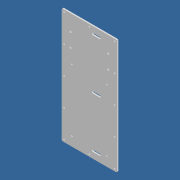
# Autodesk Inventor part: Contorller_Mount
Saved by Autodesk Inventor 2020 (Build 240168000, 168)
## iProperties
Created: 2021-07-15
Part Number: Contorller_Mount
Material: 一般
Document SubType Name: Modeling
Designer: ken113
Density: 1 g/cm^3
Appearance: 既定
Author: ken113
Autodesk Inventor part; units mm, degrees
ref_plane "YZ Plane" through (0, 0, 0) normal (1, 0, 0) x (0, 1, 0)
ref_plane "XZ Plane" through (0, 0, 0) normal (0, 1, 0) x (-1, 0, 0)
ref_plane "XY Plane" through (0, 0, 0) normal (0, 0, 1) x (1, 0, 0)
sketch "スケッチ1" plane through (0, 0, 0) normal (0, 0, 1) x (1, 0, 0)
  line L0 (50, -115) -> (-50, -115)
  line L1 (-50, -115) -> (-50, 115)
  line L2 (-50, 115) -> (50, 115)
  line L3 (50, 115) -> (50, -115)
  line L4 (50, -115) -> (-50, 115) construction
  line L5 (-50, -115) -> (50, 115) construction
  point P0 (0, 0)
  dimension "d0" = 230
  dimension "d1" = 100
  constraints: 12 end point, 2 midpoint, 2 parallel, 1 horizontal, 1 perpendicular
  measures "d0" distance of L0.end L1.end
  measures "d1" distance of L1.end L2.end
extrude "押し出し1" add sketch "スケッチ1" along normal blind 3
sketch "スケッチ2" plane through (0, 0, 3) normal (0, 0, 1) x (1, 0, 0)
  line L0 (38, -105) -> (-38, -105)
  line L1 (-38, -105) -> (-38, 30)
  line L2 (-38, 30) -> (38, 30)
  line L3 (38, 30) -> (38, -105)
  line L4 (38, -105) -> (-38, 30) construction
  line L5 (-38, -105) -> (38, 30) construction
  line L6 (-50, -115) -> (50, -115) projected
  point P0 (0, 0)
  point P1 (0, -37.5)
  point P2 (0, -37.5)
  dimension "d4" = 76
  dimension "d5" = 135
  dimension "d6" = 10
  constraints: 12 end point, 3 midpoint, 2 parallel, 1 horizontal, 1 perpendicular, 1 vertical alignment
  measures "d4" distance of L1.end L2.end
  measures "d5" distance of L2.end L0.start
  measures "d6" distance between parallel lines of L0 L6
hole "穴1" at (-38, -105, 3) at (38, -105, 3) at (38, 30, 3) at (-38, 30, 3) direction (0, 0, -1) diameter 3.2 end through all
sketch "スケッチ3" plane through (0, 0, 3) normal (0, 0, 1) x (1, 0, 0)
  line L0 (41, 60) -> (-41, 60)
  line L1 (-41, 60) -> (-41, 90)
  line L2 (-41, 90) -> (41, 90)
  line L3 (41, 90) -> (41, 60)
  line L4 (41, 60) -> (-41, 90) construction
  line L5 (-41, 60) -> (41, 90) construction
  circle A0 centre (-38, 30) radius 1.6 projected
  point P0 (0, 0)
  point P1 (0, 75)
  dimension "d14" = 82
  dimension "d15" = 30
  dimension "d16" = 30
  constraints: 12 end point, 2 midpoint, 2 parallel, 1 horizontal, 1 perpendicular
  measures "d14" distance of L1.end L2.end
  measures "d15" distance of L2.end L0.start
  measures "d16" distance from line of L0 A0.centre
hole "穴2" at (-41, 60, 3) at (41, 60, 3) at (41, 90, 3) at (-41, 90, 3) direction (0, 0, -1) diameter 4.2 end through all
sketch "スケッチ4" plane through (0, 0, 3) normal (0, 0, 1) x (1, 0, 0)
  circle A0 centre (41, 90) radius 2.1 projected
  circle A1 centre (-41, 60) radius 2.1 projected
  circle A2 centre (41, 60) radius 2.1 projected
  circle A3 centre (-41, 90) radius 2.1 projected
  circle A4 centre (38, 30) radius 1.6 projected
  circle A5 centre (-38, -105) radius 1.6 projected
  circle A6 centre (38, -105) radius 1.6 projected
  circle A7 centre (-38, 30) radius 1.6 projected
  line L0 (50, 115) -> (-50, 115) projected
  line L1 (-50, 115) -> (-50, -115) projected
  line L2 (-50, -115) -> (50, -115) projected
  line L3 (50, -115) -> (50, 115) projected
  line L4 (-60, -125) -> (-60, 125)
  line L5 (-60, 125) -> (60, 125)
  line L6 (60, 125) -> (60, -125)
  line L7 (60, -125) -> (-60, -125)
  point P0 (0, 0)
  dimension "d24" = 10
  constraints: 8 end point, 3 other
  measures "d24" distance between parallel lines of L1 L4
extrude "押し出し2" add sketch "スケッチ4" against normal up to surface (3 mm away) contours L4 L5 L6 L7
sketch "スケッチ5" plane through (0, 0, 3) normal (0, 0, 1) x (1, 0, 0)
  line L0 (60, 125) -> (-60, 125) projected
  line L1 (-60, 125) -> (-60, -125) projected
  line L2 (-60, -125) -> (60, -125) projected
  line L3 (60, -125) -> (60, 125) projected
  circle A0 centre (41, 90) radius 2.1 projected
  circle A1 centre (-41, 60) radius 2.1 projected
  circle A2 centre (41, 60) radius 2.1 projected
  circle A3 centre (-41, 90) radius 2.1 projected
  circle A4 centre (38, 30) radius 1.6 projected
  circle A5 centre (-38, -105) radius 1.6 projected
  circle A6 centre (38, -105) radius 1.6 projected
  circle A7 centre (-38, 30) radius 1.6 projected
  line L4 (-55, -120) -> (-55, 120)
  line L5 (-55, 120) -> (55, 120)
  line L6 (55, 120) -> (55, -120)
  line L7 (55, -120) -> (-55, -120)
  point P0 (0, 0)
  point P1 (0, -120)
  point P2 (0, 120)
  point P3 (55, 0)
  point P4 (55, -60)
  point P5 (-55, -60)
  point P6 (-55, 60)
  point P7 (55, 60)
  point P8 (-55, 0)
  dimension "d27" = 5
  dimension "d28" = 60
  dimension "d29" = 60
  constraints: 8 end point, 4 coincident, 4 midpoint, 4 point on line, 2 horizontal alignment, 3 other
  measures "d27" distance between parallel lines of L1 L4
  measures "d28" distance of point (-55, 60) point (-55, 0)
  measures "d29" distance of point (-55, -60) point (-55, -120)
hole "穴3" at (-55, -120, 3) at (55, -120, 3) at (0, -120, 3) at (0, 120, 3) at (-55, 120, 3) at (55, 120, 3) at (55, 0, 3) at (55, -60, 3) at (-55, -60, 3) at (-55, 60, 3) at (55, 60, 3) at (-55, 0, 3) direction (0, 0, -1) diameter 3.2 end through all
fillet "フィレット1" radius 2 4 edges at (-60, -125, 1.5) (60, -125, 1.5) (60, 125, 1.5) (-60, 125, 1.5)
sketch "スケッチ6" plane through (0, 0, 3) normal (0, 0, 1) x (1, 0, 0)
  circle A0 centre (55, 60) radius 1.6 projected
  circle A1 centre (-55, -60) radius 1.6 projected
  circle A2 centre (55, 0) radius 1.6 projected
  circle A3 centre (-55, 120) radius 1.6 projected
  circle A4 centre (0, -120) radius 1.6 projected
  circle A5 centre (-55, -120) radius 1.6 projected
  circle A6 centre (55, -120) radius 1.6 projected
  circle A7 centre (0, 120) radius 1.6 projected
  circle A8 centre (55, 120) radius 1.6 projected
  circle A9 centre (55, -60) radius 1.6 projected
  circle A10 centre (-55, 60) radius 1.6 projected
  circle A11 centre (-55, 0) radius 1.6 projected
  arc A12 (-58, 125) -> (-60, 123) centre (-58, 123) ccw projected
  line L0 (-60, 123) -> (-60, -123) projected
  arc A13 (-60, -123) -> (-58, -125) centre (-58, -123) ccw projected
  line L1 (-58, -125) -> (58, -125) projected
  arc A14 (58, -125) -> (60, -123) centre (58, -123) ccw projected
  line L2 (60, -123) -> (60, 123) projected
  arc A15 (60, 123) -> (58, 125) centre (58, 123) ccw projected
  line L3 (58, 125) -> (-58, 125) projected
  circle A16 centre (41, 90) radius 2.1 projected
  circle A17 centre (-41, 60) radius 2.1 projected
  circle A18 centre (41, 60) radius 2.1 projected
  circle A19 centre (-41, 90) radius 2.1 projected
  circle A20 centre (38, 30) radius 1.6 projected
  circle A21 centre (-38, -105) radius 1.6 projected
  circle A22 centre (38, -105) radius 1.6 projected
  circle A23 centre (-38, 30) radius 1.6 projected
  line L4 (22.5, 0) -> (7.5, 0) construction
  line L5 (22.5, 2.1) -> (7.5, 2.1)
  line L6 (7.5, -2.1) -> (22.5, -2.1)
  arc A24 (22.5, -2.1) -> (22.5, 2.1) centre (22.5, 0) ccw
  arc A25 (7.5, 2.1) -> (7.5, -2.1) centre (7.5, 0) ccw
  line L7 (22.5, -110) -> (7.5, -110) construction
  line L8 (22.5, -107.9) -> (7.5, -107.9)
  line L9 (7.5, -112.1) -> (22.5, -112.1)
  arc A26 (22.5, -112.1) -> (22.5, -107.9) centre (22.5, -110) ccw
  arc A27 (7.5, -107.9) -> (7.5, -112.1) centre (7.5, -110) ccw
  line L10 (22.5, 110) -> (7.5, 110) construction
  line L11 (22.5, 107.9) -> (7.5, 107.9)
  line L12 (7.5, 112.1) -> (22.5, 112.1)
  arc A28 (22.5, 107.9) -> (22.5, 112.1) centre (22.5, 110) ccw
  arc A29 (7.5, 112.1) -> (7.5, 107.9) centre (7.5, 110) ccw
  point P0 (15, 0)
  point P1 (15, -110)
  point P2 (15, 110)
  dimension "d38" = 4.2
  dimension "d39" = 4.2
  dimension "d40" = 4.2
  dimension "d41" = 110
  dimension "d42" = 110
  dimension "d43" = 15
  dimension "d46" = 45
  constraints: 24 end point, 12 point on circle, 12 tangent, 6 centre point, 5 parallel, 4 vertical alignment, 3 midpoint, 1 horizontal, 1 horizontal alignment
  measures "d38" distance between parallel lines of L5 L6
  measures "d39" distance between parallel lines of L8 L9
  measures "d40" distance between parallel lines of L12 L11
  measures "d41" distance of point (15, -110) point (15, 0)
  measures "d42" distance of point (15, 110) point (15, 0)
  measures "d43" distance of L7.start L7.end
  measures "d46" distance from line of point (15, 0) L2
extrude "押し出し3" cut sketch "スケッチ6" against normal blind 3 contours A24 L6 A25 L5 | A26 L9 A27 L8 | L11 A29 L12 A28
